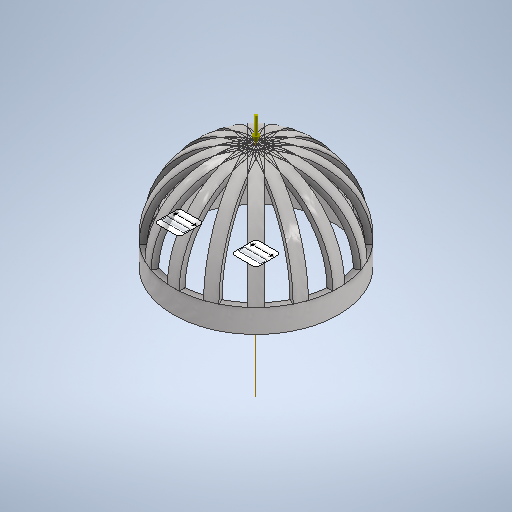
# Autodesk Inventor part: Dome
Saved by Autodesk Inventor 2025.1 (Build 291241000, 241)
## iProperties
Created: 2024-11-09
Part Number: Dome
Material: Steel, Mild, Welded
Document SubType Name: Modeling
Designer: monos
Density: 7.85 g/cm^3
Appearance: Weld - Steel Mild
Mass: 645.845 g
Surface Area: 503.286 cm^2
Volume: 82.2732 cm^3
Author: monos
Autodesk Inventor part; units mm, degrees
sketch "Sketch1" plane through (0, 0, 0) normal (0, 1, 0) x (-1, 0, 0)
  circle A0 centre (0, 0) radius 90
  circle A1 centre (0, 0) radius 83.65
  dimension "base_outer_d" = 180
  dimension "base_inner_d" = 167.3
  constraints: 2 centre point, 2 coincident
  measures "base_outer_d" diameter of A0
  measures "base_inner_d" diameter of A1
extrude "Extrusion1" add sketch "Sketch1" along normal blind 25.4
sketch "Sketch3" plane through (0, 0, 0) normal (1, 0, 0) x (0, 1, 0)
  line L0 (25.4, -90) -> (25.4, 90) projected
  arc A0 (115.4, 0) -> (25.4, 90) centre (25.4, 0) ccw
  line L1 (25.4, 0) -> (115.4, 0) construction
  line L2 (25.4, 0) -> (25.4, 90) construction
  arc A1 (109.05, 0) -> (25.4, 83.65) centre (25.4, 0) ccw
  arc A2 (25.4, -90) -> (115.4, 0) centre (25.4, 0) ccw
  arc A3 (25.4, -83.65) -> (109.05, 0) centre (25.4, 0) ccw
  line L3 (115.4, 0) -> (109.05, 0)
  line L4 (25.4, 90) -> (25.4, 83.65)
  line L5 (25.4, -90) -> (25.4, -83.65)
  line L6 (115.4, 0) -> (109.05, 0)
  point P0 (0, 0)
  point P1 (25.4, 83.65)
  dimension "d5" = 90
  dimension "d6" = 83.65
  dimension "d7" = 83.65
  constraints: 12 end point, 8 point on circle, 4 centre point, 4 collinear, 3 coincident, 3 point on line, 1 midpoint
  measures "d5" angle of L1 L2
  measures "d6" radius of A1
  measures "d7" radius of A3
extrude "Extrusion2" add sketch "Sketch3" along normal mid plane 12.7 contours L0 A3 L3 A2 | L3 A1 L0 A0
sketch "Sketch4" plane through (0, 0, 0) normal (0, 0, 1) x (1, 0, 0)
  line L0 (90, 25.4) -> (-90, 25.4) projected
  arc A0 (0, 115.4) -> (-90, 25.4) centre (0, 25.4) ccw
  arc A1 (0, 109.05) -> (-83.65, 25.4) centre (0, 25.4) ccw
  line L1 (-90, 25.4) -> (-83.65, 25.4)
  line L2 (0, 115.4) -> (0, 109.05)
  arc A2 (90, 25.4) -> (0, 115.4) centre (0, 25.4) ccw
  arc A3 (83.65, 25.4) -> (0, 109.05) centre (0, 25.4) ccw
  line L3 (0, 115.4) -> (0, 109.05)
  line L4 (83.65, 25.4) -> (90, 25.4)
  line L5 (90, 25.4) -> (83.65, 25.4)
  line L6 (-83.65, 25.4) -> (-90, 25.4)
  line L7 (0, 115.4) -> (0, 109.05)
  point P0 (0, 0)
  dimension "d8" = 83.65
  dimension "d9" = 83.65
  constraints: 14 end point, 8 point on circle, 4 centre point, 4 collinear, 3 coincident, 2 point on line, 1 horizontal, 1 midpoint, 1 perpendicular, 1 vertical
  measures "d8" radius of A1
  measures "d9" radius of A3
extrude "Extrusion3" add sketch "Sketch4" along normal mid plane 12.7 contours L0 A3 L2 A2 | L2 A1 L0 A0
ref_plane "Work Plane19" through (0, 0, 0) normal (0.7071, 0, -0.7071) x (0, 1, 0)
sketch "Sketch12" plane through (0, 0, 0) normal (0.7071, 0, -0.7071) x (0, 1, 0)
  line L0 (25.4, 59.1495) -> (25.4, -59.1495) projected
  line L1 (25.4, -90) -> (25.4, -67.9711) projected
  arc A0 (25.4, -90) -> (115.4, 0) centre (25.4, 0) ccw
  arc A1 (25.4, -83.6422) -> (109.0422, 0) centre (25.4, 0) ccw
  line L2 (25.4, -83.6422) -> (25.4, -90)
  arc A2 (115.4, 0) -> (25.4, 90) centre (25.4, 0) ccw
  line L3 (25.4, 0) -> (115.4, 0) construction
  line L4 (25.4, 0) -> (25.4, 90) construction
  line L5 (25.4, 67.9711) -> (25.4, 90) projected
  arc A3 (109.0422, 0) -> (25.4, 83.6422) centre (25.4, 0) ccw
  line L6 (25.4, 0) -> (109.0422, 0) construction
  line L7 (25.4, 0) -> (25.4, 83.6422) construction
  line L8 (25.4, 90) -> (25.4, 83.6422)
  point P0 (0, 0)
  point P1 (25.4, -83.6422)
  point P2 (115.4, 0)
  point P3 (109.0422, 0)
  dimension "d46" = 83.6422
  dimension "d50" = 90
  dimension "d51" = 83.6422
  dimension "d52" = 90
  constraints: 12 end point, 9 point on circle, 4 centre point, 3 coincident, 2 collinear, 1 midpoint, 1 point on line
  measures "d46" radius of A1
  measures "d50" angle of L3 L4
  measures "d51" radius of A3
  measures "d52" angle of L6 L7
extrude "Extrusion11" add sketch "Sketch12" along normal mid plane 12.7
ref_plane "Work Plane23" through (0, 0, 0) normal (-0.7071, 0, -0.7071) x (0, -1, 0)
sketch "Sketch14" plane through (0, 0, 0) normal (-0.7071, 0, -0.7071) x (0, -1, 0)
  line L0 (-25.4, 0) -> (-25.4, -6.35) projected
  ellipse E0 centre (-25.4, 0) end of major axis (-25.4, 217.2792) minor radius 90 (-115.3616, 6.35) -> (-115.4, 0) ccw projected
  line L1 (-25.4, -67.9711) -> (-25.4, -90) projected
  arc A0 (-115.4, 0) -> (-25.4, -90) centre (-25.4, 0) ccw
  arc A1 (-109.0422, 0) -> (-25.4, -83.6422) centre (-25.4, 0) ccw
  line L2 (-25.4, 90) -> (-25.4, 67.9711) projected
  arc A2 (-25.4, 90) -> (-115.4, 0) centre (-25.4, 0) ccw
  arc A3 (-25.4, 83.6422) -> (-109.0422, 0) centre (-25.4, 0) ccw
  line L3 (-25.4, -90) -> (-25.4, -83.6422)
  line L4 (-25.4, 83.6422) -> (-25.4, 90)
  point P0 (0, 0)
  point P1 (-109.0422, 0)
  point P2 (-25.4, 83.6422)
  dimension "d53" = 83.6422
  dimension "d54" = 83.6422
  constraints: 8 point on circle, 4 centre point, 4 end point, 3 coincident, 2 collinear, 1 other
  measures "d53" radius of A1
  measures "d54" radius of A3
ref_plane "Work Plane24" through (0, 0, 0) normal (0.3827, 0, -0.9239) x (0, -1, 0)
sketch "Sketch15" plane through (0, 0, 0) normal (0.3827, 0, -0.9239) x (0, -1, 0)
  arc A0 (-115.4, 0) -> (-25.4, -90) centre (-25.4, 0) ccw
  arc A1 (-109.0422, 0) -> (-25.4, -83.6422) centre (-25.4, 0) ccw
  arc A2 (-25.4, 90) -> (-115.4, 0) centre (-25.4, 0) ccw
  arc A3 (-25.4, 83.6422) -> (-109.0422, 0) centre (-25.4, 0) ccw
  line L0 (-25.4, -90) -> (-25.4, -83.6422)
  line L1 (-25.4, 83.6422) -> (-25.4, 90)
  point P0 (0, 0)
  point P1 (-109.0422, 0)
  dimension "d57" = 83.6422
  dimension "d58" = 83.6422
  constraints: 8 point on circle, 4 centre point, 4 end point, 3 coincident, 1 collinear
  measures "d57" radius of A1
  measures "d58" radius of A3
ref_plane "Work Plane25" through (0, 0, 0) normal (0.9239, 0, -0.3827) x (0, -1, 0)
ref_plane "Work Plane26" through (0, 0, 0) normal (0.9239, 0, 0.3827) x (0, -1, 0)
ref_plane "Work Plane27" through (0, 0, 0) normal (-0.3827, 0, -0.9239) x (0, -1, 0)
extrude "Extrusion12" add sketch "Sketch14" along normal mid plane 12.7
extrude "Extrusion13" add sketch "Sketch15" along normal mid plane 12.7
sketch "Sketch16" plane through (0, 0, 0) normal (0.9239, 0, -0.3827) x (0, -1, 0)
  arc A0 (-115.4, 0) -> (-25.4, -90) centre (-25.4, 0) ccw
  arc A1 (-109.0422, 0) -> (-25.4, -83.6422) centre (-25.4, 0) ccw
  arc A2 (-25.4, 90) -> (-115.4, 0) centre (-25.4, 0) ccw
  arc A3 (-25.4, 83.6422) -> (-109.0422, 0) centre (-25.4, 0) ccw
  line L0 (-25.4, -90) -> (-25.4, -83.6422)
  line L1 (-25.4, 83.6422) -> (-25.4, 90)
  point P0 (0, 0)
  point P1 (-109.0422, 0)
  dimension "d61" = 83.6422
  dimension "d62" = 83.6422
  constraints: 8 point on circle, 4 centre point, 4 end point, 3 coincident, 1 collinear
  measures "d61" radius of A1
  measures "d62" radius of A3
sketch "Sketch17" plane through (0, 0, 0) normal (0.9239, 0, 0.3827) x (0, -1, 0)
  arc A0 (-115.4, 0) -> (-25.4, -90) centre (-25.4, 0) ccw
  arc A1 (-109.0422, 0) -> (-25.4, -83.6422) centre (-25.4, 0) ccw
  arc A2 (-25.4, 90) -> (-115.4, 0) centre (-25.4, 0) ccw
  arc A3 (-25.4, 83.6422) -> (-109.0422, 0) centre (-25.4, 0) ccw
  line L0 (-25.4, -90) -> (-25.4, -83.6422)
  line L1 (-25.4, 83.6422) -> (-25.4, 90)
  point P0 (0, 0)
  point P1 (-109.0422, 0)
  dimension "d63" = 83.6422
  dimension "d64" = 83.6422
  constraints: 8 point on circle, 4 centre point, 4 end point, 3 coincident, 1 collinear
  measures "d63" radius of A1
  measures "d64" radius of A3
sketch "Sketch18" plane through (0, 0, 0) normal (-0.3827, 0, -0.9239) x (0, -1, 0)
  arc A0 (-115.4, 0) -> (-25.4, -90) centre (-25.4, 0) ccw
  arc A1 (-109.0422, 0) -> (-25.4, -83.6422) centre (-25.4, 0) ccw
  arc A2 (-25.4, 90) -> (-115.4, 0) centre (-25.4, 0) ccw
  arc A3 (-25.4, 83.6422) -> (-109.0422, 0) centre (-25.4, 0) ccw
  line L0 (-25.4, -90) -> (-25.4, -83.6422)
  line L1 (-25.4, 83.6422) -> (-25.4, 90)
  point P0 (0, 0)
  point P1 (-109.0422, 0)
  dimension "d65" = 83.6422
  dimension "d66" = 83.6422
  constraints: 8 point on circle, 4 centre point, 4 end point, 3 coincident, 1 collinear
  measures "d65" radius of A1
  measures "d66" radius of A3
extrude "Extrusion14" add sketch "Sketch16" along normal mid plane 12.7
extrude "Extrusion15" add sketch "Sketch17" along normal mid plane 12.7
extrude "Extrusion16" add sketch "Sketch18" along normal mid plane 12.7
body "Solid1"
